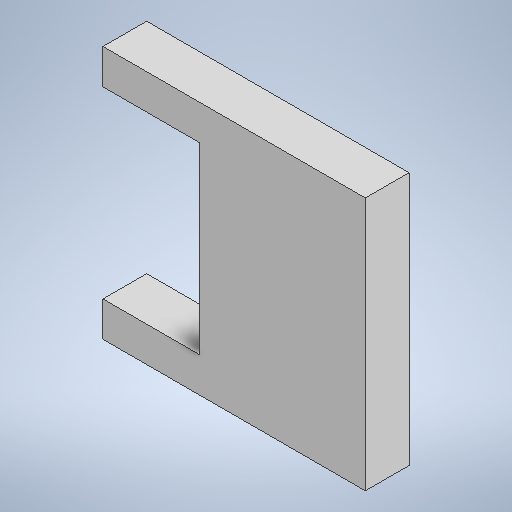
# Autodesk Inventor part: RobotBase
Saved by Autodesk Inventor 2025.3 (Build 293356000, 356)
## iProperties
Created: 2025-04-27
Part Number: RobotBase
Material: 일반
Document SubType Name: Modeling
Designer: SEON
Density: 1 g/cm^3
Appearance: 기본값
Author: SEON
Autodesk Inventor part; units mm, degrees
ref_plane "YZ Plane" through (0, 0, 0) normal (1, 0, 0) x (0, 1, 0)
ref_plane "XZ Plane" through (0, 0, 0) normal (0, 1, 0) x (-1, 0, 0)
ref_plane "XY Plane" through (0, 0, 0) normal (0, 0, 1) x (1, 0, 0)
sketch "스케치1" plane through (0, 0, 0) normal (0, 0, 1) x (1, 0, 0)
  line L0 (0, 0) -> (300, 0)
  line L1 (300, 0) -> (300, 290)
  line L2 (300, 290) -> (0, 290)
  line L3 (0, 290) -> (0, 0)
  line L4 (300, 270) -> (245, 270)
  line L5 (245, 270) -> (245, 165)
  line L6 (245, 165) -> (300, 165)
  line L7 (300, 165) -> (300, 270)
  line L8 (150, 290) -> (150, 145)
  line L9 (0, 270) -> (55, 270)
  line L10 (55, 270) -> (55, 165)
  line L11 (55, 165) -> (0, 165)
  line L12 (300, 145) -> (170.2907, 145)
  line L13 (300, 20) -> (245, 20)
  line L14 (245, 20) -> (245, 125)
  line L15 (245, 125) -> (300, 125)
  line L16 (55, 125) -> (0, 125)
  line L17 (55, 20) -> (55, 125)
  line L18 (0, 20) -> (55, 20)
  line L19 (0, 145) -> (150, 145)
  point P0 (300, 165)
  point P1 (0, 165)
  dimension "d0" = 290
  dimension "d1" = 300
  dimension "d12" = 105
  dimension "d13" = 55
  dimension "d14" = 20
  constraints: 40 end point, 12 symmetric about line, 4 horizontal, 4 parallel, 3 midpoint, 2 perpendicular, 1 point on line, 1 vertical
  measures "d0" distance of L2.end L0.start
  measures "d1" distance of L0.start L0.end
  measures "d12" distance of L4.end L5.end
  measures "d13" distance of L5.end L6.end
  measures "d14" distance between parallel lines of L2 L4
extrude "돌출1" add sketch "스케치1" along normal blind 25 contours L3 L11 L10 L9 L2 L8 L19
